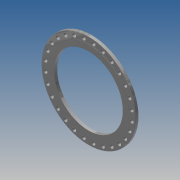
# Autodesk Inventor part: A1-19027-500-01 32in CL150 RF flange
Saved by Autodesk Inventor 2017.3 (Build 213257000, 257)
## iProperties
Created: 2016-02-11
Part Number: A1-19027-500-01 32in CL150 RF flange
Material: Steel, Mild
Document SubType Name: Modeling
Designer: Graeme_Van_Dongen
Density: 7.85 g/cm^3
Appearance: Steel
Description: 32" CLASS 150 B16.47 Ser.A RFBL FLANGE, A350 LF2
Mass: 100198 g
Surface Area: 10597.9 cm^2
Volume: 12764.1 cm^3
Author: Graeme_Van_Dongen
Autodesk Inventor part; units mm, degrees
ref_plane "YZ Plane" through (0, 0, 0) normal (1, 0, 0) x (0, 1, 0)
ref_plane "XZ Plane" through (0, 0, 0) normal (0, 1, 0) x (-1, 0, 0)
ref_plane "XY Plane" through (0, 0, 0) normal (0, 0, 1) x (1, 0, 0)
sketch "Sketch1" plane through (0, 0, 0) normal (0, 0, 1) x (1, 0, 0)
  circle A0 centre (0, 0) radius 530.225
  circle A1 centre (0, 0) radius 387.35
  dimension "d0" = 1060.45
  dimension "d1" = 774.7
  constraints: 2 centre point, 2 coincident
  measures "d0" diameter of A0
  measures "d1" diameter of A1
extrude "Extrusion1" add sketch "Sketch1" along normal blind 33.3375
sketch "Sketch2" plane through (0, 0, 33.3375) normal (0, 0, 1) x (1, 0, 0)
  line L0 (-485.8756, -54.745) -> (485.8756, 54.745)
  line L1 (-485.8756, -54.745) -> (492.0244, -54.745) construction
  point P0 (0, 0)
  point P1 (0, 0)
  dimension "d4" = 977.9
  dimension "d5" = 6.429
  constraints: 4 end point, 2 coincident, 1 equal length, 1 horizontal, 1 midpoint
  measures "d4" distance of L0.start L0.end
  measures "d5" angle of L1 L0
hole "Hole1" at (485.8756, 54.745, 33.3375) direction (0, 0, -1) diameter 41.275 end through all
chamfer "Chamfer1" distance 0.7937 angle 45 2 edges at (485.8756, 75.3825, 33.3375) (485.8756, 75.3825, 0)
pattern_circular "Circular Pattern1" count 28 over 360 about axis through (0, 0, -10) along (0, 0, 1) of "Hole1", "Chamfer1"
chamfer "Chamfer2" distance 1.5875 angle 45 2 edges at (-530.225, 0, 33.3375) (-530.225, 0, 0)
chamfer "Chamfer4" distance 0.7937 angle 45 1 edges at (-387.35, 0, 0)
sketch "Sketch4" plane through (0, 0, 33.3375) normal (0, 0, 1) x (1, 0, 0)
  circle A0 centre (0, 0) radius 387.35 projected
  circle A1 centre (0, 0) radius 457.2
  dimension "d31" = 914.4
  constraints: 1 centre point, 1 coincident
  measures "d31" diameter of A1
extrude "Extrusion3" add sketch "Sketch4" along normal blind 1.5875
body "Solid1"
